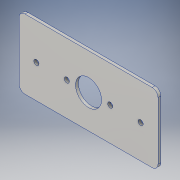
# Autodesk Inventor part: GearboxPlate
Saved by Autodesk Inventor 2016 (Build 200138000, 138)
## iProperties
Created: 2017-01-19
Part Number: GearboxPlate
Material: Aluminum 6061
Document SubType Name: Modeling
Designer: Kyle
Density: 2.7 g/cm^3
Appearance: Aluminum - Flat
Mass: 92.9085 g
Surface Area: 236.019 cm^2
Volume: 34.4106 cm^3
Author: Kyle
Autodesk Inventor part; units mm, degrees
ref_plane "YZ Plane" through (0, 0, 0) normal (1, 0, 0) x (0, 1, 0)
ref_plane "XZ Plane" through (0, 0, 0) normal (0, 1, 0) x (-1, 0, 0)
ref_plane "XY Plane" through (0, 0, 0) normal (0, 0, 1) x (1, 0, 0)
sketch "Sketch1" plane through (0, 0, 0) normal (0, 0, 1) x (1, 0, 0)
  line L0 (0, 0) -> (152.4, 0)
  line L1 (152.4, 0) -> (152.4, 76.2)
  line L2 (152.4, 76.2) -> (0, 76.2)
  line L3 (0, 76.2) -> (0, 0)
  dimension "d0" = 152.4
  dimension "d1" = 76.2
  constraints: 8 end point, 2 parallel, 1 horizontal, 1 perpendicular
  measures "d0" distance of L2.end L1.end
  measures "d1" distance of L1.end L0.end
extrude "Extrusion1" add sketch "Sketch1" along normal blind 3.175
sketch "Sketch2" plane through (0, 0, 3.175) normal (0, 0, 1) x (1, 0, 0)
  line L0 (152.4, 76.2) -> (0, 76.2) projected
  line L1 (0, 76.2) -> (0, 0) projected
  circle A0 centre (52.3875, 36.5125) radius 2.8067
  circle A1 centre (100.0125, 36.5125) radius 2.8067
  circle A2 centre (19.05, 36.5125) radius 2.8067
  circle A3 centre (133.35, 36.5125) radius 2.8067
  circle A4 centre (76.2, 36.5125) radius 14.2875
  line L2 (0, 0) -> (152.4, 0) projected
  dimension "d8" = 5.6134
  dimension "d9" = 5.6134
  dimension "d11" = 5.6134
  dimension "d12" = 5.6134
  dimension "d22" = 28.575
  dimension "d23" = 76.2
  dimension "d24" = 36.5125
  dimension "d25" = 36.5125
  dimension "d26" = 36.5125
  dimension "d27" = 36.5125
  dimension "d28" = 36.5125
  constraints: 5 centre point
  measures "d8" diameter of A0
  measures "d9" diameter of A1
  measures "d11" diameter of A2
  measures "d12" diameter of A3
  measures "d22" diameter of A4
  measures "d23" distance from line of L1 A4.centre
  measures "d24" distance from line of L2 A4.centre
  measures "d25" distance from line of L2 A0.centre
  measures "d26" distance from line of L2 A2.centre
  measures "d27" distance from line of L2 A1.centre
  measures "d28" distance from line of L2 A3.centre
extrude "Extrusion3" cut sketch "Sketch2" against normal blind 25.4
fillet "Fillet2" radius 6.35 4 edges at (152.4, 0, 1.5875) (152.4, 76.2, 1.5875) (0, 76.2, 1.5875) (0, 0, 1.5875)
body "Solid1"
